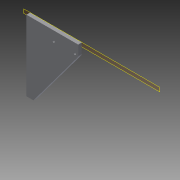
# Autodesk Inventor part: support
Saved by Autodesk Inventor 2013 (Build 170138000, 138)
## iProperties
Created: 2013-07-23
Part Number: support
Material: Generic
Document SubType Name: Modeling
Designer: employee
Density: 1 g/cm^3
Author: employee
Autodesk Inventor part; units mm, degrees
ref_plane "YZ Plane" through (0, 0, 0) normal (1, 0, 0) x (0, 1, 0)
ref_plane "XZ Plane" through (0, 0, 0) normal (0, 1, 0) x (-1, 0, 0)
ref_plane "XY Plane" through (0, 0, 0) normal (0, 0, 1) x (1, 0, 0)
ref_plane "Work Plane1" through (0, 0, 0) normal (0, 0, 1) x (1, 0, 0)
sketch "Sketch1" plane through (0, 0, 0) normal (0, 0, 1) x (1, 0, 0)
  circle A0 centre (95.734, -21) radius 4.05 projected
  circle A1 centre (170.734, -21) radius 4.05 projected
  line L0 (78.234, -5) -> (78.234, 0) projected
  arc A2 (83.234, -10) -> (78.234, -5) centre (78.234, -10) ccw projected
  line L1 (83.234, -10) -> (83.234, -21) projected
  arc A3 (83.234, -21) -> (108.234, -21) centre (95.734, -21) ccw projected
  line L2 (108.234, -21) -> (108.234, -10) projected
  arc A4 (113.234, -5) -> (108.234, -10) centre (113.234, -10) ccw projected
  line L3 (113.234, -5) -> (153.234, -5) projected
  arc A5 (158.234, -10) -> (153.234, -5) centre (153.234, -10) ccw projected
  line L4 (158.234, -10) -> (158.234, -21) projected
  arc A6 (158.234, -21) -> (183.234, -21) centre (170.734, -21) ccw projected
  line L5 (183.234, -21) -> (183.234, -10) projected
  arc A7 (188.234, -5) -> (183.234, -10) centre (188.234, -10) ccw projected
  line L6 (188.234, 0) -> (188.234, -5) projected
  line L7 (78.234, 0) -> (188.234, 0) projected
  line L8 (437.5, 12.7) -> (437.5, 0) projected
  line L9 (0, 12.7) -> (437.5, 12.7) projected
  line L10 (0, 0) -> (0, 12.7) projected
  line L11 (437.5, 0) -> (0, 0) projected
  line L12 (0, 12.7) -> (0, -237.3)
  line L13 (0, -237.3) -> (25, -237.3)
  line L14 (25, -237.3) -> (180.7539, -28.4734)
  line L15 (183.234, -10) -> (183.234, 12.7)
  line L16 (183.234, 12.7) -> (0, 12.7)
  dimension "d0" = 25
  dimension "d2" = 250
  constraints: 10 end point, 3 perpendicular, 2 tangent, 1 collinear, 1 point on circle, 1 point on line
  measures "d0" distance of L12.end L13.end
  measures "d2" distance of L9.start L12.end
extrude "Extrusion1" add sketch "Sketch1" along normal blind 12.7 contours A2 L1 A3 L2 A4 L3 A5 L4 A6 L14 L13 L12 L11 L0 | L0 L7 L15 L5 A6 L4 A5 L3 A4 L2 A3 L1 A2 | L11 L10 L9 L15 L7
body "Solid1"
